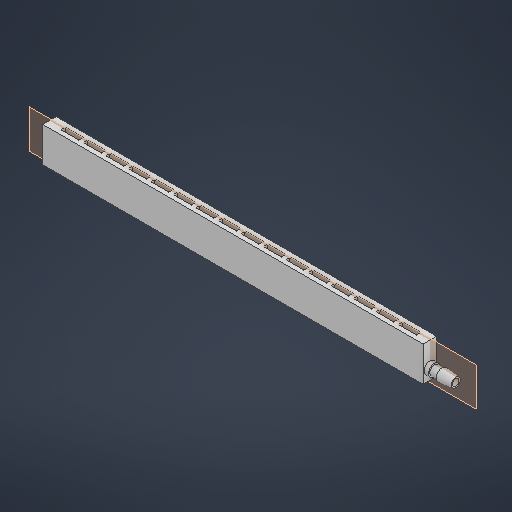
# Autodesk Inventor part: Sprinkler
Saved by Autodesk Inventor 2026.2 (Build 302298010, 298A)
## iProperties
Created: 2026-06-09
Part Number: Sprinkler
Material: Genérico
Document SubType Name: Modeling
Designer: pauli
Density: 1 g/cm^3
Appearance: Padrão
Author: pauli
Autodesk Inventor part; units mm, degrees
ref_plane "YZ Plane" through (0, 0, 0) normal (1, 0, 0) x (0, 1, 0)
ref_plane "XZ Plane" through (0, 0, 0) normal (0, 1, 0) x (-1, 0, 0)
ref_plane "XY Plane" through (0, 0, 0) normal (0, 0, 1) x (1, 0, 0)
sketch "Esboço1" plane through (0, 0, 0) normal (0, 0, 1) x (1, 0, 0)
  line L0 (0, 0) -> (153, 0)
  line L1 (153, 0) -> (153, 5.8)
  line L2 (153, 5.8) -> (0, 5.8)
  line L3 (0, 5.8) -> (0, 0)
  dimension "d0" = 153
  dimension "d1" = 5.8
  constraints: 8 end point, 2 parallel, 1 horizontal, 1 perpendicular
  measures "d0" distance of L2.end L1.end
  measures "d1" distance of L1.end L0.end
extrude "Extrusão1" add sketch "Esboço1" along normal blind 3
sketch "Esboço2" plane through (0, 0, 3) normal (0, 0, 1) x (1, 0, 0)
  line L0 (0, 5.8) -> (0, 0) projected
  line L1 (0, 2.9) -> (-8, 2.9) construction
  line L2 (-8, 2.9) -> (-8, 14.4)
  line L3 (-8, 2.9) -> (-8, -1.1)
  line L4 (153, 0) -> (153, 5.8) projected
  line L5 (153, 2.9) -> (161, 2.9) construction
  line L6 (161, 2.9) -> (161, 14.4)
  line L7 (161, 2.9) -> (161, -1.1)
  line L8 (161, 14.4) -> (-8, 14.4)
  line L9 (-8, -1.1) -> (161, -1.1)
  dimension "d4" = 8
  dimension "d5" = 11.5
  dimension "d6" = 4
  dimension "d7" = 8
  dimension "d8" = 11.5
  dimension "d9" = 4
  constraints: 16 end point, 3 vertical, 2 horizontal, 2 midpoint, 1 perpendicular
  measures "d4" distance of L1.start L1.end
  measures "d5" distance of L1.end L2.end
  measures "d6" distance of L1.end L3.end
  measures "d7" distance of L5.start L5.end
  measures "d8" distance of L5.end L6.end
  measures "d9" distance of L5.end L7.end
extrude "Extrusão2" add sketch "Esboço2" along normal blind 2
sketch "Esboço3" plane through (0, 0, 5) normal (0, 0, 1) x (1, 0, 0)
  line L0 (161, 14.4) -> (-8, 14.4) projected
  line L1 (-8, 14.4) -> (-2, 14.4)
  line L2 (-2, 14.4) -> (-2, 2.4)
  line L3 (-2, 2.4) -> (161, 2.4)
  line L4 (161, -1.1) -> (161, 14.4) projected
  line L5 (161, 2.4) -> (161, -1.1)
  line L6 (161, -1.1) -> (-8, -1.1)
  line L7 (-8, -1.1) -> (-8, 14.4)
  point P0 (0, 0)
  dimension "d12" = 6
  dimension "d13" = 12
  dimension "d14" = 90
  dimension "d15" = 90
  constraints: 12 end point, 3 perpendicular, 2 point on line, 1 collinear
  measures "d12" distance of L0.end L1.end
  measures "d13" distance of L1.end L2.end
  measures "d14" angle of L1 L2
  measures "d15" angle of L3 L2
extrude "Extrusão3" add sketch "Esboço3" along normal blind 2 contours L2 L3 L4 L6 L7 L0
sketch "Esboço4" plane through (0, 0, 5) normal (0, 0, 1) x (1, 0, 0)
  line L0 (-2, 2.4) -> (161, 2.4) projected
  line L1 (-2, 2.4) -> (6, 2.4) construction
  line L2 (6, 2.4) -> (6, 14.4)
  line L3 (6, 14.4) -> (8, 14.4)
  line L4 (8, 14.4) -> (8, 2.4)
  line L5 (8, 2.4) -> (6, 2.4)
  line L6 (8, 2.4) -> (16, 2.4) construction
  line L7 (16, 2.4) -> (16, 14.4)
  line L8 (16, 14.4) -> (18, 14.4)
  line L9 (18, 14.4) -> (18, 2.4)
  line L10 (18, 2.4) -> (16, 2.4)
  line L11 (18, 2.4) -> (26, 2.4) construction
  line L12 (26, 2.4) -> (26, 14.4)
  line L13 (26, 14.4) -> (28, 14.4)
  line L14 (28, 14.4) -> (28, 2.4)
  line L15 (28, 2.4) -> (26, 2.4)
  line L16 (28, 2.4) -> (36, 2.4) construction
  line L17 (36, 2.4) -> (36, 14.4)
  line L18 (36, 14.4) -> (38, 14.4)
  line L19 (38, 14.4) -> (38, 2.4)
  line L20 (38, 2.4) -> (36, 2.4)
  line L21 (38, 2.4) -> (46, 2.4) construction
  line L22 (46, 2.4) -> (46, 14.4)
  line L23 (46, 14.4) -> (48, 14.4)
  line L24 (48, 14.4) -> (48, 2.4)
  line L25 (48, 2.4) -> (46, 2.4)
  line L26 (48, 2.4) -> (56, 2.4) construction
  line L27 (56, 2.4) -> (56, 14.4)
  line L28 (56, 14.4) -> (58, 14.4)
  line L29 (58, 14.4) -> (58, 2.4)
  line L30 (58, 2.4) -> (56, 2.4)
  line L31 (58, 2.4) -> (66, 2.4) construction
  line L32 (66, 2.4) -> (66, 14.4)
  line L33 (66, 14.4) -> (68, 14.4)
  line L34 (68, 14.4) -> (68, 2.4)
  line L35 (68, 2.4) -> (66, 2.4)
  line L36 (68, 2.4) -> (76, 2.4) construction
  line L37 (76, 2.4) -> (76, 14.4)
  line L38 (76, 14.4) -> (78, 14.4)
  line L39 (78, 14.4) -> (78, 2.4)
  line L40 (78, 2.4) -> (76, 2.4)
  line L41 (78, 2.4) -> (86, 2.4) construction
  line L42 (86, 2.4) -> (86, 14.4)
  line L43 (86, 14.4) -> (88, 14.4)
  line L44 (88, 14.4) -> (88, 2.4)
  line L45 (88, 2.4) -> (86, 2.4)
  line L46 (88, 2.4) -> (96, 2.4) construction
  line L47 (96, 2.4) -> (96, 14.4)
  line L48 (96, 14.4) -> (98, 14.4)
  line L49 (98, 14.4) -> (98, 2.4)
  line L50 (98, 2.4) -> (96, 2.4)
  line L51 (98, 2.4) -> (106, 2.4) construction
  line L52 (106, 2.4) -> (106, 14.4)
  line L53 (106, 14.4) -> (108, 14.4)
  line L54 (108, 14.4) -> (108, 2.4)
  line L55 (108, 2.4) -> (106, 2.4)
  line L56 (108, 2.4) -> (116, 2.4) construction
  line L57 (116, 2.4) -> (116, 14.4)
  line L58 (116, 14.4) -> (118, 14.4)
  line L59 (118, 14.4) -> (118, 2.4)
  line L60 (118, 2.4) -> (116, 2.4)
  line L61 (118, 2.4) -> (126, 2.4) construction
  line L62 (126, 2.4) -> (126, 14.4)
  line L63 (126, 14.4) -> (128, 14.4)
  line L64 (128, 14.4) -> (128, 2.4)
  line L65 (128, 2.4) -> (126, 2.4)
  line L66 (128, 2.4) -> (136, 2.4) construction
  line L67 (136, 2.4) -> (136, 14.4)
  line L68 (136, 14.4) -> (138, 14.4)
  line L69 (138, 14.4) -> (138, 2.4)
  line L70 (138, 2.4) -> (136, 2.4)
  line L71 (138, 2.4) -> (146, 2.4) construction
  line L72 (146, 2.4) -> (146, 14.4)
  line L73 (146, 14.4) -> (148, 14.4)
  line L74 (148, 14.4) -> (148, 2.4)
  line L75 (148, 2.4) -> (146, 2.4)
  line L76 (148, 2.4) -> (156, 2.4) construction
  line L77 (156, 2.4) -> (156, 14.4)
  line L78 (156, 14.4) -> (158, 14.4)
  line L79 (158, 14.4) -> (158, 2.4)
  line L80 (158, 2.4) -> (156, 2.4)
  line L81 (158, 2.4) -> (162, 2.4) construction
  point P0 (0, 0)
  point P1 (10, 0)
  point P2 (20, 0)
  point P3 (30, 0)
  point P4 (40, 0)
  point P5 (50, 0)
  point P6 (60, 0)
  point P7 (70, 0)
  point P8 (80, 0)
  point P9 (90, 0)
  point P10 (100, 0)
  point P11 (110, 0)
  point P12 (120, 0)
  point P13 (130, 0)
  point P14 (140, 0)
  point P15 (150, 0)
  point P16 (146, 2.4)
  point P17 (148, 2.4)
  point P18 (16, 2.4)
  point P19 (138, 2.4)
  point P20 (116, 2.4)
  point P21 (108, 2.4)
  point P22 (96, 2.4)
  point P23 (68, 2.4)
  point P24 (86, 2.4)
  point P25 (88, 2.4)
  point P26 (76, 2.4)
  point P27 (158, 2.4)
  dimension "d18" = 8
  dimension "d19" = 12
  dimension "d20" = 2
  dimension "d21" = 12
  dimension "d22" = 90
  dimension "d25" = 10
  dimension "d30" = 4
  constraints: 162 end point, 90 horizontal alignment, 45 collinear, 30 parallel, 2 perpendicular, 1 vertical, 3 other
  measures "d18" distance of L1.start L1.end
  measures "d19" distance of L1.end L2.end
  measures "d20" distance of L2.end L3.end
  measures "d21" distance of L3.end L4.end
  measures "d22" angle of L3 L4
  measures "d25" distance of point (0, 0) point (10, 0)
  measures "d30" distance of L79.end L81.end
extrude "Extrusão4" add sketch "Esboço4" along normal blind 2
sketch "Esboço5" plane through (158, 2.4, 5) normal (1, 0, 0) x (0, 0, -1)
  line L0 (-2, 0) -> (0, 0) projected
  line L1 (0, 0) -> (0, 12) projected
  line L2 (-1.75, 1.5) -> (-0.0833, 11.5)
  line L3 (0, 12) -> (0, 0)
  line L4 (-2, 0) -> (0, 0)
  line L5 (-2, 0) -> (-1.75, 0)
  line L6 (-1.75, 0) -> (-1.75, 1.5)
  line L7 (0, 0) -> (0, 12) projected
  line L8 (0, 12) -> (0, 11.5)
  line L9 (0, 11.5) -> (-0.0833, 11.5)
  point P0 (5, -2.4)
  point P1 (-1.75, 0)
  dimension "d33" = 0.25
  dimension "d38" = 0.5
  constraints: 14 end point, 2 perpendicular, 2 point on line, 1 collinear, 1 vertical
  measures "d33" distance of L0.start L5.end
  measures "d38" distance of L1.end L8.end
extrude "Extrusão5" cut sketch "Esboço5" against normal up to surface (152 mm away)
sketch "Esboço6" plane through (0, 0, 7) normal (0, 0, 1) x (1, 0, 0)
  line L0 (-8, -1.1) -> (161, -1.1) projected
  line L1 (161, 14.4) -> (-8, 14.4) projected
  line L2 (-8, -1.1) -> (-8, 14.4)
  line L3 (-8, 14.4) -> (161, 14.4)
  line L4 (161, 14.4) -> (161, -1.1)
  line L5 (161, -1.1) -> (-8, -1.1)
  point P0 (0, 0)
  constraints: 8 end point, 2 perpendicular, 1 collinear, 1 vertical
extrude "Extrusão6" add sketch "Esboço6" along normal blind 2
sketch "Esboço7" plane through (161, -1.1, 3) normal (1, 0, 0) x (0, 0, -1)
  line L0 (-2, 3.5) -> (-4, 3.5) projected
  line L1 (-3, 3.5) -> (-3, 6.4) construction
  circle A0 centre (-3, 4.95) radius 1.45
  circle A1 centre (-3, 4.95) radius 2
  point P0 (3, 1.1)
  dimension "d39" = 2.9
  dimension "d40" = 4
  constraints: 2 end point, 2 midpoint, 1 centre point, 1 coincident, 1 vertical, 1 vertical alignment, 2 other
  measures "d39" distance of L1.start L1.end
  measures "d40" diameter of A1
extrude "Extrusão7" add sketch "Esboço7" along normal blind 11.5
sketch "Esboço8" plane through (158, 13.9, 5) normal (1, 0, 0) x (0, 0, -1)
  line L0 (-1.75, -11.5) -> (-2, -11.5) projected
  line L1 (0, 0.5) -> (0, -11.5) projected
  line L2 (-2, -8.3179) -> (-2, 0.5) projected
  line L3 (0, 0.5) -> (-2, 0.5) projected
  line L4 (-1, 0.5) -> (-1, -11.5) construction
  line L5 (0, -11.5) -> (-2, -11.5) projected
  line L6 (-2, -11.5) -> (-1, -8.7525)
  line L7 (-2, -11.5) -> (1.5599, -11.5) construction
  line L8 (0, -11.5) -> (-1, -8.7525)
  line L9 (-2, -11.5) -> (-2, -8.5597)
  line L10 (-2, -8.5597) -> (0, -8.5597)
  line L11 (0, -8.5597) -> (0, -11.5)
  point P0 (5, -13.9)
  dimension "d44" = 12
  dimension "d45" = 70
  constraints: 14 end point, 2 perpendicular, 2 point on line, 2 vertical, 1 horizontal, 1 midpoint
  measures "d44" distance of L4.start L4.end
  measures "d45" angle of L7 L6
extrude "Extrusão8" add sketch "Esboço8" along normal up to surface (3 mm away) contours L9 L10 L1 L8 L6
sketch "Esboço9" plane through (158, 5.3403, 6.5099) normal (0, 1, 0) x (1, 0, 0)
  line L0 (3, -0.4901) -> (3, -2.4901) projected
  line L1 (3, 1.3991) -> (3, 1.5099) projected
  line L2 (3, -0.4901) -> (3, 1.5099)
  line L3 (3, 1.5099) -> (-0.0308, 1.5099)
  line L4 (-0.0308, 1.5099) -> (-0.0308, -0.4901)
  line L5 (-0.0308, -0.4901) -> (3, -0.4901)
  point P0 (-158, 6.5099)
  constraints: 8 end point, 3 perpendicular, 1 vertical
extrude "Extrusão9" add sketch "Esboço9" along normal up to surface (9.0597 mm away)
ref_plane "Plano de trabalho1" through (0, 0, 6) normal (0, 0, 1) x (1, 0, 0)
sketch "Esboço10" plane through (0, 0, 6) normal (0, 0, 1) x (1, 0, 0)
  line L0 (172.5, 1.85) -> (172.5, 5.85) projected
  line L1 (172.5, 5.85) -> (166.4, 5.85)
  line L2 (161, 5.85) -> (172.5, 5.85) projected
  line L3 (172.5, 3.85) -> (166.4, 3.85)
  line L4 (166.4, 5.85) -> (166.4, 6.45)
  line L5 (166.4, 6.45) -> (172.5, 5.85)
  point P0 (0, 0)
  dimension "d50" = 6.1
  dimension "d51" = 2.6
  constraints: 8 end point, 1 horizontal, 1 midpoint, 1 perpendicular, 1 point on line
  measures "d50" distance of L1.end L0.end
  measures "d51" distance of L3.end L4.end
revolve "Revolução1" add sketch "Esboço10" angle 360 about axis through (172.5, 3.85, 6) along (-1, 0, 0)
sketch "Esboço11" plane through (161, -1.1, 3) normal (1, 0, 0) x (0, 0, -1)
  point P0 (3, 1.1)
sketch "Esboço12" plane through (161, -1.1, 3) normal (1, 0, 0) x (0, 0, -1)
  circle A0 centre (-3, 4.95) radius 2 projected
  circle A1 centre (-3, 4.95) radius 2
  circle A2 centre (-3, 4.95) radius 2.6
  point P0 (3, 1.1)
  dimension "d53" = 5.2
  constraints: 2 centre point, 2 coincident
  measures "d53" diameter of A2
extrude "Extrusão10" add sketch "Esboço12" along normal blind 2
